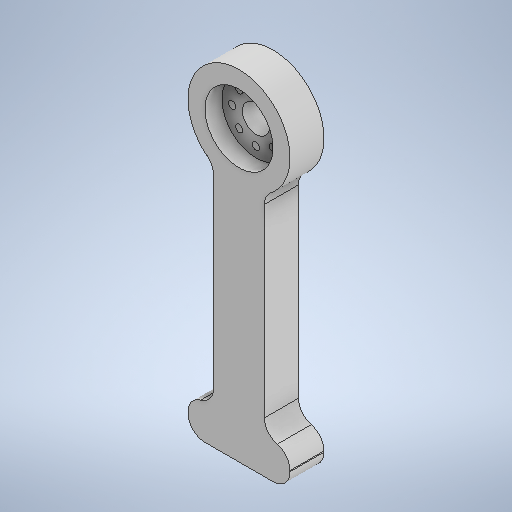
# Autodesk Inventor part: bearing_bracket3
Saved by Autodesk Inventor 2026.1 (Build 301233000, 233)
## iProperties
Created: 2026-04-11
Part Number: bearing_bracket3
Material: Generic
Document SubType Name: Modeling
Designer: chris
Density: 1 g/cm^3
Appearance: Default
Author: chris
Autodesk Inventor part; units mm, degrees
ref_plane "YZ Plane" through (0, 0, 0) normal (1, 0, 0) x (0, 1, 0)
ref_plane "XZ Plane" through (0, 0, 0) normal (0, 1, 0) x (-1, 0, 0)
ref_plane "XY Plane" through (0, 0, 0) normal (0, 0, 1) x (1, 0, 0)
sketch "Sketch1" plane through (0, 0, 0) normal (0, 0, 1) x (1, 0, 0)
  circle A0 centre (0, 0) radius 30
  dimension "d0" = 60
  constraints: 1 centre point, 1 coincident
  measures "d0" diameter of A0
extrude "Extrusion1" add sketch "Sketch1" along normal blind 5
sketch "Sketch2" plane through (0, 0, 5) normal (0, 0, 1) x (1, 0, 0)
  circle A0 centre (0, 0) radius 24.95
  dimension "d3" = 49.9
  constraints: 1 centre point, 1 coincident
  measures "d3" diameter of A0
extrude "Extrusion2" add sketch "Sketch2" along normal blind 5
sketch "Sketch3" plane through (0, 0, 10) normal (0, 0, 1) x (1, 0, 0)
  circle A0 centre (0, 0) radius 15
  dimension "d6" = 30
  constraints: 1 centre point, 1 coincident
  measures "d6" diameter of A0
extrude "Extrusion3" cut sketch "Sketch3" against normal through all
sketch "Sketch4" plane through (0, 0, 0) normal (0, 0, -1) x (-1, 0, 0)
  circle A0 centre (0, 0) radius 20
  dimension "d9" = 40
  constraints: 1 centre point, 1 coincident
  measures "d9" diameter of A0
extrude "Extrusion4" add sketch "Sketch4" against normal blind 5
sketch "Sketch5" plane through (0, 0, 0) normal (0, 0, -1) x (-1, 0, 0)
  circle A0 centre (0, 0) radius 3.5
  dimension "d12" = 7
  constraints: 1 centre point, 1 coincident
  measures "d12" diameter of A0
extrude "Extrusion5" cut sketch "Sketch5" against normal through all
sketch "Sketch6" plane through (0, 0, 5) normal (0, 0, 1) x (1, 0, 0)
  circle A0 centre (7, 0) radius 1.05
  point P0 (0, 0)
  dimension "d15" = 2.1
  dimension "d16" = 7
  constraints: 1 centre point
  measures "d15" diameter of A0
  measures "d16" distance of point (0, 0) A0.centre
extrude "Extrusion6" cut sketch "Sketch6" against normal through all
pattern_circular "Circular Pattern1" count 8 over 360 about axis through (0, 0, -10) along (0, 0, 1) of "Extrusion6"
sketch "Sketch9" plane through (0, 0, 0) normal (0, 0, -1) x (-1, 0, 0)
  circle A0 centre (0, 0) radius 15
  circle A1 centre (-4.9497, -4.9497) radius 1.05 projected
  circle A2 centre (0, -7) radius 1.05 projected
  circle A3 centre (4.9497, -4.9497) radius 1.05 projected
  circle A4 centre (7, 0) radius 1.05 projected
  circle A5 centre (4.9497, 4.9497) radius 1.05 projected
  circle A6 centre (0, 7) radius 1.05 projected
  circle A7 centre (-4.9497, 4.9497) radius 1.05 projected
  circle A8 centre (-7, 0) radius 1.05 projected
  circle A9 centre (0, 0) radius 3.5 projected
  circle A10 centre (0, 0) radius 30 projected
  dimension "d35" = 30
  constraints: 1 centre point, 1 coincident
  measures "d35" diameter of A0
extrude "Extrusion9" cut sketch "Sketch9" against normal through all contours A10
sketch "Sketch10" plane through (0, 0, 5) normal (0, 0, 1) x (1, 0, 0)
  circle A0 centre (0, 0) radius 10
  circle A1 centre (4.9497, -4.9497) radius 1.05 projected
  circle A2 centre (0, -7) radius 1.05 projected
  circle A3 centre (-4.9497, -4.9497) radius 1.05 projected
  circle A4 centre (-7, 0) radius 1.05 projected
  circle A5 centre (-4.9497, 4.9497) radius 1.05 projected
  circle A6 centre (0, 7) radius 1.05 projected
  circle A7 centre (4.9497, 4.9497) radius 1.05 projected
  circle A8 centre (7, 0) radius 1.05 projected
  circle A9 centre (0, 0) radius 3.5 projected
  circle A10 centre (0, 0) radius 15 projected
  dimension "d38" = 20
  constraints: 1 centre point, 1 coincident
  measures "d38" diameter of A0
extrude "Extrusion10" add sketch "Sketch10" along normal blind 5 contours A10
sketch "Sketch11" plane through (0, 0, 0) normal (0, 0, -1) x (-1, 0, 0)
  line L0 (-7.5, 0) -> (7.5, 0)
  line L1 (7.5, 0) -> (7.5, -80)
  line L2 (7.5, -80) -> (-7.5, -80)
  line L3 (-7.5, -80) -> (-7.5, 0)
  line L4 (-7.5, 0) -> (7.5, -80) construction
  line L5 (7.5, 0) -> (-7.5, -80) construction
  circle A0 centre (0, 0) radius 15 projected
  circle A1 centre (-4.9497, -4.9497) radius 1.05 projected
  circle A2 centre (0, -7) radius 1.05 projected
  circle A3 centre (4.9497, -4.9497) radius 1.05 projected
  circle A4 centre (7, 0) radius 1.05 projected
  circle A5 centre (4.9497, 4.9497) radius 1.05 projected
  circle A6 centre (0, 7) radius 1.05 projected
  circle A7 centre (-4.9497, 4.9497) radius 1.05 projected
  circle A8 centre (-7, 0) radius 1.05 projected
  circle A9 centre (0, 0) radius 3.5 projected
  line L6 (-15, -75) -> (15, -75)
  line L7 (15, -75) -> (15, -85)
  line L8 (15, -85) -> (-15, -85)
  line L9 (-15, -85) -> (-15, -75)
  line L10 (-15, -75) -> (15, -85) construction
  line L11 (15, -75) -> (-15, -85) construction
  point P0 (0, -40)
  point P1 (7.5, -12.9904)
  point P2 (-7.5, -12.9904)
  point P3 (0, -80)
  point P4 (-7.5, -75)
  point P5 (7.5, -75)
  point P6 (0, 0)
  dimension "d41" = 80
  dimension "d42" = 15
  dimension "d43" = 40
  dimension "d46" = 30
  dimension "d47" = 10
  constraints: 24 end point, 6 midpoint, 4 parallel, 2 horizontal, 2 perpendicular, 1 vertical alignment
  measures "d41" distance of L0.end L1.end
  measures "d42" distance of L0.start L0.end
  measures "d43" distance of point (0, 0) point (0, -40)
  measures "d46" distance of L7.end L8.end
  measures "d47" distance of L6.end L7.end
extrude "Extrusion11" add sketch "Sketch11" against normal blind 10 contours A0 L1 L6 L3 | L6 L1 L2 L3 | L3 L2 L1 L6 L7 L8 L9
fillet "Fillet1" radius 5 8 edges at (-7.5, -12.9904, 5) (7.5, -12.9904, 5) (7.5, -75, 5) (15, -75, 5) (15, -85, 5) (-7.5, -75, 5) (-15, -75, 5) (-15, -85, 5)
sketch "Sketch12" plane through (0, 0, 5) normal (0, 0, 1) x (1, 0, 0)
  circle A0 centre (0, 0) radius 4
  dimension "d49" = 8
  constraints: 1 centre point, 1 coincident
  measures "d49" diameter of A0
extrude "Extrusion12" cut sketch "Sketch12" against normal blind 10
body "Solid1"
